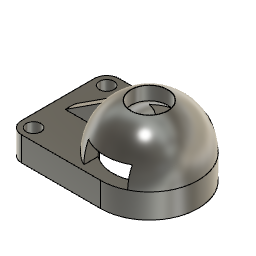
drawing_10 v1 (Autodesk Fusion 360 design; units mm, degrees)
Autodesk Fusion 360 part; units mm, degrees
note: some values were not read from the file. Set by a fixed rule: which sketch regions a step uses.
sketch "Sketch1" plane through (0, 0, 0) normal (0, 0, 1) x (1, 0, 0)
  line L0 (0, 0) -> (37.5, 0)
  line L1 (0, 0) -> (-37.5, 0)
  line L2 (-37.5, 0) -> (-37.5, 40)
  line L3 (37.5, 0) -> (37.5, -40)
  line L4 (-37.5, 40) -> (37.5, 40)
  line L5 (37.5, 40) -> (37.5, -40)
  line L6 (37.5, -40) -> (-37.5, -40)
  line L7 (-37.5, -40) -> (-37.5, 40)
  dimension "d1" = 37.5
  dimension "d2" = 37.5
  dimension "d3" = 40
  dimension "d4" = 40
  constraint coincident L0.start L1.start
  constraint horizontal L0
  constraint parallel L0 L1
  constraint perpendicular L1 L2
  constraint perpendicular L0 L3
  constraint horizontal L4
  constraint vertical L5
  constraint horizontal L6
  constraint vertical L7
  measures "d1" distance of L0.start L0.end
  measures "d2" distance of L0.start L1.end
  measures "d3" distance of L1.end L2.end
  measures "d4" distance of L0.end L3.end
extrude "Extrude1" add sketch "Sketch1" along normal blind 20 makes body 1
sketch "Sketch2" plane through (0, 0, 20) normal (0, 0, 1) x (-1, 0, 0)
  line L0 (37.5, 40) -> (-37.5, 40)
  line L1 (-37.5, 40) -> (-37.5, -40)
  line L2 (-37.5, -40) -> (37.5, -40)
  line L3 (37.5, -40) -> (37.5, 40)
  line L4 (37.5, 0) -> (37.5, -30)
  line L5 (37.5, 0) -> (37.5, 30)
  line L6 (-37.5, -40) -> (27.5, -40)
  circle A0 centre (27.5, -30) radius 6
  circle A1 centre (27.5, 30) radius 6
  point P0 (37.5, 0)
  dimension "d8" = 30
  dimension "d10" = 12
  dimension "d11" = 12
  constraint coincident P0 L4.start
  constraint perpendicular L2 L4
  constraint parallel L3 L5
  constraint coincident L1.end L2.start
  constraint perpendicular L1 L6
  measures "d8" distance of P0 L5.end
  measures "d10" diameter of A0
  measures "d11" diameter of A1
extrude "Extrude2" cut sketch "Sketch2" against normal blind 90 contours A0 | A1 bodies 1
sketch "Sketch3" plane through (0, 0, 20) normal (0, 0, 1) x (-1, 0, 0)
  circle A0 centre (27.5, 30) radius 6
  circle A1 centre (27.5, -30) radius 6
  line L0 (37.5, 40) -> (-37.5, 40)
  line L1 (-37.5, 40) -> (-37.5, -40)
  line L2 (-37.5, -40) -> (37.5, -40)
  line L3 (37.5, -40) -> (37.5, 40)
  circle A2 centre (27.5, 30) radius 10
  circle A3 centre (27.5, -30) radius 10
  dimension "d14" = 20
  dimension "d15" = 20
  constraint concentric A0 A2
  constraint concentric A1 A3
  measures "d14" diameter of A2
  measures "d15" diameter of A3
extrude "Extrude3" cut sketch "Sketch3" against normal blind 35 contours L0 L3 A2 | L2 L3 A3 bodies 1
sketch "Sketch4" plane through (0, 0, 20) normal (0, 0, 1) x (-1, 0, 0)
  arc A0 (37.5, 30) -> (27.5, 40) centre (27.5, 30) ccw
  line L0 (27.5, 40) -> (-37.5, 40)
  line L1 (-37.5, 40) -> (-37.5, -40)
  line L2 (-37.5, -40) -> (27.5, -40)
  arc A1 (27.5, -40) -> (37.5, -30) centre (27.5, -30) ccw
  line L3 (37.5, -30) -> (37.5, 30)
  circle A2 centre (27.5, 30) radius 6
  circle A3 centre (27.5, -30) radius 6
  circle A4 centre (-37.5, 0) radius 40
  dimension "d18" = 80
  constraint midpoint L1 A4.centre
  measures "d18" diameter of A4
extrude "Extrude4" add sketch "Sketch4" against normal blind 20 contours L1 A4 | L1 A4 bodies 1
sketch "Sketch5" plane through (0, 0, 0) normal (0, 0, -1) x (1, 0, 0)
  line L0 (37.5, 40) -> (-27.5, 40)
  arc A0 (-27.5, 40) -> (-37.5, 30) centre (-27.5, 30) ccw
  line L1 (-37.5, 30) -> (-37.5, -30)
  arc A1 (-37.5, -30) -> (-27.5, -40) centre (-27.5, -30) ccw
  line L2 (-27.5, -40) -> (37.5, -40)
  arc A2 (37.5, -40) -> (37.5, 40) centre (37.5, 0) ccw
  circle A3 centre (-27.5, 30) radius 6
  circle A4 centre (-27.5, -30) radius 6
  point P0 (37.5, 0)
  constraint coincident P0 A2.centre
sphere "SpherePrimitive1" add diameter 80 placed x (-1, 0, 0) y (0, -1, 0) z (0, 0, 1) at (37.5, 0, 20) bodies 1
extrude "Extrude5" cut sketch "Sketch5" along normal blind 20 bodies 1
sketch "Sketch7" plane through (0, 0, 0) normal (0, 0, -1) x (1, 0, 0)
  line L0 (37.5, 40) -> (-27.5, 40)
  arc A0 (-27.5, 40) -> (-37.5, 30) centre (-27.5, 30) ccw
  line L1 (-37.5, 30) -> (-37.5, -30)
  arc A1 (-37.5, -30) -> (-27.5, -40) centre (-27.5, -30) ccw
  line L2 (-27.5, -40) -> (37.5, -40)
  arc A2 (37.5, -40) -> (37.5, 40) centre (37.5, 0) ccw
  circle A3 centre (-27.5, 30) radius 6
  circle A4 centre (-27.5, -30) radius 6
  circle A5 centre (37.5, 0) radius 30
  dimension "d24" = 60
  constraint concentric A2 A5
  measures "d24" diameter of A5
extrude "Extrude6" cut sketch "Sketch7" against normal blind 20 contours A5 bodies 1
sphere "SpherePrimitive2" cut diameter 60 placed x (1, 0, 0) y (0, -1, 0) z (0, 0, -1) at (37.5, 0, 20) bodies 1
sketch "Sketch9" plane through (0, 0, 0) normal (0, 0, 1) x (1, 0, 0)
ref_plane "WorkPlane1" through (0, 0, 57) normal (0, 0, 1) x (1, 0, 0)
sketch "Sketch10" plane through (0, 0, 57) normal (0, 0, 1) x (1, 0, 0)
  line L0 (7.4967, 46.768) -> (98.4073, 46.768)
  line L1 (98.4073, 46.768) -> (98.4073, -40.4525)
  line L2 (98.4073, -40.4525) -> (7.4967, -40.4525)
  line L3 (7.4967, -40.4525) -> (7.4967, 46.768)
  constraint horizontal L0
  constraint vertical L1
  constraint horizontal L2
  constraint vertical L3
extrude "Extrude7" cut sketch "Sketch10" along normal blind 20 bodies 1
sketch "Sketch11" plane through (0, 0, 57) normal (0, 0, 1) x (-1, 0, 0)
  circle A0 centre (-37.5, 0) radius 15.1987
  circle A1 centre (-37.5, 0) radius 15
  dimension "d31" = 30
  constraint concentric A0 A1
  measures "d31" diameter of A1
extrude "Extrude8" cut sketch "Sketch11" against normal blind 15 contours A1 bodies 1
sketch "Sketch12" plane through (0, 0, 20) normal (0, 0, 1) x (-1, 0, 0)
  arc A0 (-37.5, -40) -> (-37.5, 40) centre (-37.5, 0) ccw
  line L0 (-37.5, -40) -> (27.5, -40)
  arc A1 (27.5, -40) -> (37.5, -30) centre (27.5, -30) ccw
  line L1 (37.5, -30) -> (37.5, 30)
  arc A2 (37.5, 30) -> (27.5, 40) centre (27.5, 30) ccw
  line L2 (27.5, 40) -> (-37.5, 40)
  circle A3 centre (27.5, 30) radius 6
  circle A4 centre (27.5, -30) radius 6
  line L3 (-37.5, 40) -> (27.5, 40)
  line L4 (27.5, 0) -> (27.5, -4)
  line L5 (27.5, -4) -> (27.5, 0)
  line L6 (27.5, 0) -> (27.5, 4)
  line L7 (27.5, 4) -> (0, 4)
  line L8 (0, 4) -> (0, -4)
  line L9 (0, -4) -> (27.5, -4)
  line L10 (27.5, -4) -> (0, -4)
  line L11 (0, -4) -> (0, 4)
  line L12 (0, 4) -> (27.5, 4)
  line L13 (27.5, 4) -> (27.5, -4)
  line L14 (27.5, -4) -> (-12.731, -4)
  line L15 (-12.731, -4) -> (-12.731, 4)
  line L16 (-12.731, 4) -> (27.5, 4)
  line L17 (27.5, 4) -> (27.5, -4)
  point P0 (37.5, 0)
  dimension "d34" = 65
  dimension "d37" = 8
  constraint coincident A0.end L2.end
  constraint tangent A0 L3
  constraint midpoint L1 P0
  constraint perpendicular L6 L7
  constraint perpendicular L7 L8
  constraint perpendicular L4 L9
  constraint horizontal L10
  constraint vertical L11
  constraint horizontal L12
  constraint vertical L13
  constraint horizontal L14
  constraint vertical L15
  constraint horizontal L16
  constraint vertical L17
  measures "d34" distance of A0.end A2.end
  measures "d37" distance of L7.end L8.end
extrude "Extrude9" add sketch "Sketch12" along normal blind 26 separate body contours A0 L7 L8 L9 L10 L11 L12 L14 L16 | A0 L4 L5 L6 L7 L9 L10 L12 L13 L14 L16 L17 | L8 L11 L14 L15 L16 makes body 2
sketch "Sketch13" plane through (0, 4, 0) normal (0, 1, 0) x (-1, 0, 0)
  line L0 (-12.731, 20) -> (27.5, 20)
  line L1 (27.5, 20) -> (27.5, 46)
  line L2 (27.5, 46) -> (-12.731, 46)
  line L3 (-12.731, 46) -> (-12.731, 20)
  line L4 (-12.731, 46) -> (27.5, 20)
  constraint coincident L2.end L3.start
  constraint coincident L0.end L1.start
extrude "Extrude10" cut sketch "Sketch13" against normal blind 24 contours L1 L2 L4 bodies 2
combine "Combine1" operation add target body 2 tool bodies 1
sketch "Sketch14" plane through (-37.5, 0, 0) normal (-1, 0, 0) x (0, -1, 0)
  line L0 (30, 0) -> (30, 20)
  line L1 (30, 20) -> (-30, 20)
  line L2 (-30, 20) -> (-30, 0)
  line L3 (-30, 0) -> (30, 0)
  line L4 (0, 0) -> (-15, 0)
  line L5 (0, 0) -> (15, 0)
  line L6 (-15, 0) -> (15, 0)
  line L7 (15, 0) -> (15, 14)
  line L8 (15, 14) -> (-15, 14)
  line L9 (-15, 14) -> (-15, 0)
  dimension "d42" = 15
  dimension "d44" = 14
  constraint coincident L4.start L5.start
  constraint parallel L3 L4
  constraint parallel L3 L5
  constraint horizontal L6
  constraint vertical L7
  constraint horizontal L8
  constraint vertical L9
  measures "d42" distance of L4.start L4.end
  measures "d44" distance of L4.end L8.end
extrude "Extrude11" cut sketch "Sketch14" against normal blind 75 contours L3 L4 L5 L6 L7 L8 L9 bodies 2
sketch "Sketch15" plane through (0, -40, 0) normal (0, -1, 0) x (1, 0, 0)
  line L0 (-27.5, 20) -> (-27.5, 0)
  line L1 (-27.5, 0) -> (37.5, 0)
  line L2 (37.5, 20) -> (-27.5, 20)
  line L3 (37.5, 20) -> (37.5, 36)
  line L4 (37.5, 36) -> (55.5, 36)
  line L5 (55.5, 36) -> (37.5, 36)
  line L6 (37.5, 36) -> (19.5, 36)
  line L7 (55.5, 36) -> (55.5, 20)
  line L8 (19.5, 36) -> (55.5, 36)
  line L9 (55.5, 36) -> (55.5, 20)
  line L10 (55.5, 20) -> (19.5, 20)
  line L11 (19.5, 20) -> (19.5, 36)
  dimension "d47" = 16
  dimension "d48" = 18
  dimension "d49" = 18
  constraint coincident L2.start L3.start
  constraint perpendicular L2 L3
  constraint perpendicular L3 L4
  constraint perpendicular L3 L6
  constraint perpendicular L4 L7
  constraint horizontal L8
  constraint vertical L9
  constraint horizontal L10
  constraint vertical L11
  measures "d47" distance of L2.start L3.end
  measures "d48" distance of L3.end L4.end
  measures "d49" distance of L3.end L6.end
extrude "Extrude12" cut sketch "Sketch15" against normal blind 105 bodies 2
